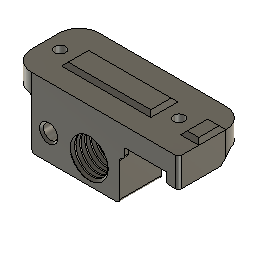
umbilical_mount (Autodesk Fusion 360 design; units mm, degrees)
Autodesk Fusion 360 part; units mm, degrees
sketch "Sketch1" plane through (0, 0, 0) normal (0, 1, 0) x (1, 0, 0)
  line L0 (0, 0) -> (26, 0)
  line L1 (26, 0) -> (26, -15)
  line L2 (26, -15) -> (0, -15)
  line L3 (0, -15) -> (0, 0)
  circle A0 centre (17, -7.5) radius 5.5
  line L4 (26, -7.5) -> (0, -7.5) construction
  circle A1 centre (5, -7.5) radius 2.1
  line L5 (24.99, -15) -> (24.99, -13.99)
  line L6 (24.99, -13.99) -> (26, -12.98)
  line L7 (0, -15) -> (-6, -15)
  line L8 (-6, -15) -> (-6, -20.6)
  line L9 (-6, -20.6) -> (43.39, -20.6)
  line L10 (43.39, -20.6) -> (43.39, -15)
  line L11 (43.39, -15) -> (26, -15)
  line L12 (43.39, -15) -> (43.39, -12)
  line L13 (42.19, -15) -> (42.19, -13.99)
  line L14 (42.19, -13.99) -> (41.18, -12.98)
  line L15 (41.18, -12.98) -> (41.18, -12)
  line L16 (41.18, -12) -> (43.39, -12)
  line L17 (41.18, -12.98) -> (41.18, -15)
  dimension "d1" = 11
  dimension "d2" = 15
  dimension "d3" = 4.2
  dimension "d4" = 12
  dimension "d5" = 5
  dimension "d6" = 26
  dimension "d33" = 1.01
  dimension "d34" = 1.01
  dimension "d35" = 135
  dimension "d36" = 6
  dimension "d37" = 5.6
  dimension "d38" = 1.2
  dimension "d39" = 135
  dimension "d40" = 1.01
  dimension "d41" = 1.01
  dimension "d42" = 3
  dimension "d43" = 17.2
  constraint horizontal L0
  constraint vertical L1
  constraint horizontal L2
  constraint vertical L3
  constraint coincident L0.start L3.end
  constraint midpoint L1 L4.start
  constraint midpoint L3 L4.end
  constraint coincident A0.centre L4
  constraint coincident L4 A1.centre
  constraint coincident L2 L5.start
  constraint perpendicular L2 L5
  constraint coincident L1 L6.end
  constraint perpendicular L3 L7
  constraint perpendicular L7 L8
  constraint perpendicular L8 L9
  constraint perpendicular L9 L10
  constraint perpendicular L10 L11
  constraint perpendicular L11 L12
  constraint coincident L11 L13.start
  constraint perpendicular L11 L13
  constraint perpendicular L11 L15
  constraint perpendicular L15 L16
  constraint coincident L11 L17.end
  constraint perpendicular L11 L17
  measures "d1" diameter of A0
  measures "d2" distance of L0.end L1.end
  measures "d3" diameter of A1
  measures "d4" distance of A0.centre A1.centre
  measures "d5" distance of L3 A1.centre
  measures "d6" distance of L0.start L0.end
  measures "d33" distance of L1 L5
  measures "d34" distance of L5.start L5.end
  measures "d35" angle of L5 L6
  measures "d36" distance of L2.end L7.end
  measures "d37" distance of L7.end L8.end
  measures "d38" distance of L12 L13
  measures "d39" angle of L13 L14
  measures "d40" distance of L13.start L13.end
  measures "d41" distance of L13 L15
  measures "d42" distance of L10.end L12.end
  measures "d43" distance of L5 L13
extrude "Extrude1" add sketch "Sketch1" along normal blind 12.5 contours L0 L1 L2 L3 L5 L6 | L2 L7 L8 L9 L10 L11 | L11 L12 L13 L14 L15 L16
thread "Thread1" "ISO Metric profile 12.0 M12x1.5 M12x1.5 6H" major diameter 12.203 minor diameter 10.526 pitch 1.5 angle 60 modelled right hand crest width 0.4065 on face at (22.4727, 4.1667, 8.0476) crest through (22.263, 0.375, 7.5)
sketch "Sketch4" plane through (0, 12.5, 0) normal (0, 1, 0) x (-1, 0, 0)
  line L0 (-42.19, 15) -> (-24.99, 15)
  line L1 (-24.99, 15) -> (-24.99, 13.99)
  line L2 (-24.99, 13.99) -> (-26, 12.98)
  line L3 (-26, 12.98) -> (-26, 0)
  line L4 (-26, 0) -> (0, 0)
  line L5 (0, 0) -> (0, 15)
  line L6 (0, 15) -> (6, 15)
  line L7 (6, 15) -> (6, 20.6)
  line L8 (6, 20.6) -> (-43.39, 20.6)
  line L9 (-43.39, 20.6) -> (-43.39, 12)
  line L10 (-43.39, 12) -> (-41.18, 12)
  line L11 (-41.18, 12) -> (-41.18, 12.98)
  line L12 (-41.18, 12.98) -> (-42.19, 13.99)
  line L13 (-42.19, 13.99) -> (-42.19, 15)
  circle A0 centre (-5, 7.5) radius 2.1
  spline S0 degree 3 poles (-21.9829, 9.1941) (-21.8118, 9.866) (-21.5093, 10.4974) (-20.6699, 11.628) (-20.1348, 12.1115) (-18.8933, 12.8604) (-18.1948, 13.1118) (-16.7206, 13.3398) (-15.9579, 13.3063) (-14.7587, 13.018) (-14.3103, 12.8507) (-13.4559, 12.4096) (-13.0537, 12.1358) (-12.6884, 11.8172) knots 0 0 0 0 0.208013 0.208013 0.422162 0.422162 0.642443 0.642443 0.868854 0.868854 1.011546 1.011546 1.156581 1.156581 1.156581 1.156581
  arc A1 (-11.1054, 9.0754) -> (-12.6884, 11.8172) centre (-17, 7.5) ccw
  spline S1 degree 3 poles (-11.1054, 9.0754) (-10.9549, 8.3074) (-10.954, 7.5177) (-11.2546, 6.0034) (-11.5455, 5.292) (-12.3755, 4.0401) (-12.8999, 3.5074) (-14.1084, 2.6879) (-14.7764, 2.4025) (-15.9041, 2.1664) (-16.3368, 2.1285) (-17.1939, 2.1576) (-17.6153, 2.2226) (-18.0243, 2.3376) knots 0 0 0 0 0.234781 0.234781 0.463418 0.463418 0.685909 0.685909 0.90225 0.90225 1.03239 1.03239 1.160187 1.160187 1.160187 1.160187
  arc A2 (-21.9829, 9.1941) -> (-18.0243, 2.3376) centre (-17, 7.5) ccw
  line L14 (6, 15) -> (-43.39, 15)
  constraint coincident L6.end L7.start
  constraint coincident L9 L14.end
  constraint perpendicular L9 L14
extrude "Extrude5" add sketch "Sketch4" along normal blind 7.5 contours L0 L6 L7 L8 L9 L14
sketch "Sketch5" plane through (0, 0, 15) normal (0, 0, -1) x (1, 0, 0)
  line L0 (42.19, 0) -> (24.99, 0)
  line L1 (24.99, 0) -> (24.99, -12.5)
  line L2 (24.99, -12.5) -> (0, -12.5)
  line L3 (0, -12.5) -> (0, 0)
  line L4 (0, 0) -> (-6, 0)
  line L5 (-6, 0) -> (-6, -20)
  line L6 (-6, -20) -> (43.39, -20)
  line L7 (43.39, -20) -> (43.39, -12.5)
  line L8 (43.39, -12.5) -> (42.19, -12.5)
  line L9 (42.19, -12.5) -> (42.19, 0)
  line L10 (-6, -10) -> (43.39, -10) construction
  line L11 (43.39, 0) -> (43.39, -12.5) construction
  line L12 (33.59, 0) -> (33.59, -20) construction
  circle A0 centre (33.59, -10) radius 1.6
  circle A1 centre (-1.6, -10) radius 1.6
  circle A2 centre (-1.6, -10) radius 3
  circle A3 centre (33.59, -10) radius 3
  line L13 (39.69, 0) -> (39.69, -1)
  line L14 (27.49, -1) -> (27.49, 0)
  line L15 (39.69, -1) -> (42.19, -1)
  line L16 (27.49, -1) -> (24.99, -1)
  dimension "d46" = 3.2
  dimension "d48" = 6
  dimension "d58" = 12.2
  dimension "d60" = 1
  constraint midpoint L5 L10.start
  constraint perpendicular L5 L10
  constraint coincident L11 L10.end
  constraint midpoint L0 L12.start
  constraint coincident L6 L12.end
  constraint perpendicular L6 L12
  constraint midpoint L12 A0.centre
  constraint equal A0 A1
  constraint tangent L3 A1
  constraint coincident L10 A1.centre
  constraint concentric A1 A2
  constraint concentric A0 A3
  constraint equal A2 A3
  constraint coincident L0 L13.start
  constraint perpendicular L0 L13
  constraint coincident L0 L14.end
  constraint perpendicular L0 L14
  constraint symmetric L12 L13 L14
  constraint equal L13 L14
  constraint coincident L9 L15.end
  constraint perpendicular L9 L15
  constraint coincident L1 L16.end
  constraint perpendicular L1 L16
  measures "d46" diameter of A0
  measures "d48" diameter of A3
  measures "d58" distance of L13.end L14.start
  measures "d60" distance of L14.start L14.end
extrude "Extrude6" cut sketch "Sketch5" against normal up to surface (5.6 mm away) contours A1 | A0
extrude "Extrude7" cut sketch "Sketch5" along normal up to surface (15 mm away) and the other way blind 3 contours L2 L3 A2 | L2 L3 A2 | A3
extrude "Extrude9" add sketch "Sketch5" along normal up to surface (3 mm away) contours L0 L9 L13 L15 | L0 L1 L14 L16
fillet "Fillet2" radius 6 3 edges at (-6, 0, 17.8) (-6, 20, 17.8) (43.39, 20, 17.8)
fillet "Fillet2" radius 1 1 edges at (43.39, 0, 16.3)
fillet "Fillet2" radius 1 1 edges at (0.0583, 12.5, 7.5)
fillet "Fillet2" radius 1 2 edges at (0, 3.7311, 15) (12.5242, 12.5, 15)
fillet "Fillet2" radius 1 3 edges at (26, 0.5, 12) (27.49, 0.5, 12) (39.69, 0.5, 12)
fillet "Fillet2" radius 0.5 2 edges at (26, 1, 12.49) (41.18, 1, 12.49)
fillet "Fillet2" radius 1 2 edges at (26, 6.25, 0) (0, 3.7311, 0)
sketch "Sketch6" plane through (0, 0, 20.6) normal (0, 0, 1) x (-1, 0, 0)
  arc A0 (-42.39, 0) -> (-43.39, -1) centre (-42.39, -1) ccw
  line L0 (-43.39, -1) -> (-43.39, -14)
  arc A1 (-43.39, -14) -> (-37.39, -20) centre (-37.39, -14) ccw
  line L1 (-37.39, -20) -> (0, -20)
  arc A2 (0, -20) -> (6, -14) centre (0, -14) ccw
  line L2 (6, -14) -> (6, -6)
  arc A3 (6, -6) -> (0, 0) centre (0, -6) ccw
  line L3 (0, 0) -> (-42.39, 0)
  circle A4 centre (1.6, -10) radius 1.6
  circle A5 centre (-33.59, -10) radius 1.6
  line L4 (6, -10) -> (-43.39, -10) construction
  line L5 (6, -6) -> (-43.39, -6)
  line L6 (-43.39, -14) -> (6, -14)
  line L7 (-2.8, -6) -> (-2.8, -14)
  line L8 (-29.19, -6) -> (-29.19, -14)
  line L9 (-37.99, -6) -> (-37.99, -14)
  dimension "d79" = 8
  dimension "d80" = 4.4
  dimension "d81" = 4.4
  dimension "d82" = 4.4
  constraint midpoint L2 L4.start
  constraint coincident L0 L4.end
  constraint perpendicular L0 L4
  constraint coincident L2 A3.start
  constraint coincident L0 L5.end
  constraint perpendicular L0 L5
  constraint coincident L0 A1.start
  constraint coincident L2 A2.end
  constraint perpendicular L2 L6
  constraint symmetric L4 L5 L6
  constraint coincident L5 L7.start
  constraint coincident L6 L7.end
  constraint perpendicular L6 L7
  constraint coincident L5 L8.start
  constraint perpendicular L5 L8
  constraint coincident L5 L9.start
  constraint coincident L6 L9.end
  constraint perpendicular L6 L9
  measures "d79" distance of L5 L6
  measures "d80" distance of A4.centre L7
  measures "d81" distance of A5.centre L8
  measures "d82" distance of A5.centre L9
extrude "Extrude10" add sketch "Sketch6" along normal blind 1 contours L0 L5 L6 L9 | L5 L6 L7 L8
chamfer "Chamfer2" distance 0.6 angle 45 2 edges at (3.0421, 0, 6.7406) (3.0421, 12.5, 6.7406)
chamfer "Chamfer2" distance 3 angle 45 1 edges at (42.79, 12.5, 15)
chamfer "Chamfer2" distance 1 angle 45 2 faces at (20.3933, 8.6667, 21.6) (39.79, 11.3333, 21.6)
equation "d34 = d33"
equation "d39 = d35"
equation "d40 = d33"
equation "d41 = d40"
equation "d44 = 20 mm - 12.5 mm"
equation "d81 = d80"
equation "d82 = d81"
